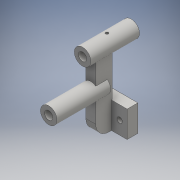
# Autodesk Inventor part: Supporto DX
Saved by Autodesk Inventor 2016 (Build 200138000, 138)
## iProperties
Created: 2016-12-03
Part Number: Supporto DX
Material: Generic
Document SubType Name: Modeling
Designer: Muhammad
Density: 1 g/cm^3
Appearance: Default
Author: Muhammad
Autodesk Inventor part; units mm, degrees
note: some values were not read from the file. Chosen so that the rebuilt part matches the saved one: direction of "Hole2".
ref_plane "YZ Plane" through (0, 0, 0) normal (1, 0, 0) x (0, 1, 0)
ref_plane "XZ Plane" through (0, 0, 0) normal (0, 1, 0) x (-1, 0, 0)
sketch "Sketch1" plane through (0, 0, 0) normal (0, 1, 0) x (-1, 0, 0)
  line L0 (3, 20.25) -> (-3, 20.25)
  line L1 (-3, 20.25) -> (-3, -20.25)
  line L2 (-3, -20.25) -> (3, -20.25)
  line L3 (3, -20.25) -> (3, 20.25)
  line L4 (3, 20.25) -> (-3, -20.25) construction
  line L5 (-3, 20.25) -> (3, -20.25) construction
  point P0 (0, 0)
  dimension "d0" = 6
  dimension "d1" = 40.5
  constraints: 12 end point, 2 midpoint, 2 parallel, 1 horizontal, 1 perpendicular
  measures "d0" distance of L2.end L1.end
  measures "d1" distance of L1.end L0.end
extrude "Extrusion1" add sketch "Sketch1" along normal blind 10
fillet "Fillet1" radius 8 1 edges at (0, 0, -20.25)
sketch "Sketch2" plane through (0, 10, 0) normal (0, 1, 0) x (1, 0, 0)
  line L0 (3, 20.25) -> (-3, 20.25) construction
  line L1 (0, 20.25) -> (0, -24.25) construction
  circle A0 centre (0, -24.25) radius 5
  point P0 (0, 0)
  dimension "d5" = 44.5
  dimension "d6" = 10
  constraints: 2 end point, 1 centre point, 1 coincident, 1 midpoint, 1 vertical
  measures "d5" distance of L1.start L1.end
  measures "d6" diameter of A0
extrude "Extrusion2" add sketch "Sketch2" along normal blind 14.5 and the other way blind 15
sketch "Sketch3" plane through (0, 0, 0) normal (0, -1, 0) x (1, 0, 0)
  line L0 (3, -20.25) -> (-3, -20.25) construction
  line L1 (0, -20.25) -> (0, 3.75) construction
  circle A0 centre (0, 3.75) radius 5
  point P0 (0, 0)
  dimension "d11" = 24
  dimension "d12" = 10
  constraints: 2 end point, 1 centre point, 1 coincident, 1 midpoint, 1 vertical
  measures "d11" distance of L1.start L1.end
  measures "d12" diameter of A0
extrude "Extrusion3" add sketch "Sketch3" along normal blind 25.5 and the other way blind 7
sketch "Sketch4" plane through (0, 10, 0) normal (0, 1, 0) x (1, 0, 0)
  line L0 (-3, 20.25) -> (3, 20.25) construction
  line L1 (0, 20.25) -> (0, 12.25) construction
  line L2 (-12.5, 4.25) -> (12.5, 4.25)
  line L3 (12.5, 4.25) -> (12.5, 20.25)
  line L4 (12.5, 20.25) -> (-12.5, 20.25)
  line L5 (-12.5, 20.25) -> (-12.5, 4.25)
  line L6 (-12.5, 4.25) -> (12.5, 20.25) construction
  line L7 (12.5, 4.25) -> (-12.5, 20.25) construction
  point P0 (0, 0)
  dimension "d17" = 8
  dimension "d18" = 25
  constraints: 14 end point, 3 midpoint, 2 parallel, 1 horizontal, 1 perpendicular, 1 vertical
  measures "d17" distance of L1.start L1.end
  measures "d18" distance of L4.end L3.end
extrude "Extrusion4" add sketch "Sketch4" along normal blind 6 and the other way blind 0.5
sketch "Sketch5" plane through (0, 16, 0) normal (0, 1, 0) x (1, 0, 0)
  line L0 (-3, 20.25) -> (3, 20.25) construction
  line L1 (0, 20.25) -> (0, 12.25) construction
  line L2 (0, 12.25) -> (-8, 12.25) construction
  circle A0 centre (-8, 12.25) radius 1.6
  circle A1 centre (8, 12.25) radius 1.6
  point P0 (0, 0)
  dimension "d23" = 8
  dimension "d24" = 8
  dimension "d25" = 3.2
  constraints: 4 end point, 2 centre point, 1 coincident, 1 midpoint, 1 perpendicular, 1 symmetric about line, 1 vertical, 1 other
  measures "d23" distance of L1.start L1.end
  measures "d24" distance of L1.end L2.end
  measures "d25" diameter of A0
extrude "Extrusion5" cut sketch "Sketch5" against normal through all
sketch "Sketch6" plane through (0, 24.5, 24.25) normal (0, 1, 0) x (1, 0, 0)
  circle A0 centre (0, 0) radius 2.5
  point P0 (0, 24.25)
  dimension "d28" = 5
  constraints: 1 centre point
  measures "d28" diameter of A0
extrude "Extrusion6" cut sketch "Sketch6" against normal through all
sketch "Sketch7" plane through (0, -25.5, 3.75) normal (0, -1, 0) x (1, 0, 0)
  circle A0 centre (0, 0) radius 1.3196
  point P0 (0, -3.75)
  constraints: 1 centre point
hole "Hole1" at (0, -25.5, 3.75) direction (0, 1, 0) diameter 5 depth 13 tip angle 118
ref_plane "Work Plane1" through (0, 0, 29.25) normal (0, 0, 1) x (1, 0, 0)
sketch "Sketch8" plane through (0, 0, 29.25) normal (0, 0, 1) x (1, 0, 0)
  line L0 (5, 24.5) -> (-5, 24.5) projected
  line L1 (0, 24.5) -> (0, 9.75)
  circle A0 centre (0, 9.75) radius 0.8
  point P0 (0, 0)
  dimension "d39" = 14.75
  dimension "d40" = 1.6
  constraints: 2 end point, 1 centre point, 1 coincident, 1 midpoint, 1 vertical
  measures "d39" distance of L1.start L1.end
  measures "d40" diameter of A0
hole "Hole2" at (0, 9.75, 29.25) direction (0, 0, -1) diameter 1.6 end up to surface countersink diameter 1.7 countersink angle 45
body "Solid1"
